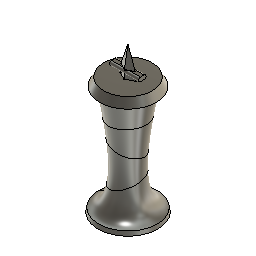
King_v2.4 (Autodesk Fusion 360 design; units mm, degrees)
Autodesk Fusion 360 part; units mm, degrees
sketch "Sketch1" plane through (0, 0, 0) normal (0, 1, 0) x (1, 0, 0)
  spline S0 degree 5 poles (-36.0949, 0) (-34.6298, -0.4528) (-31.8391, -1.6025) (-28.072, -4.0591) (-23.9013, -8.8233) (-20.1701, -17.3686) (-17.9602, -28.572) (-17.1934, -42.2972) (-17.719, -58.2807) (-19.3724, -76.2348) (-22.0047, -95.8993) (-24.8041, -112.843) (-27.2642, -126.1805) (-29.0618, -135.3476) (-30, -140) knots 0 0 0 0 0 0 0.1 0.2 0.3 0.4 0.5 0.6 0.7 0.8 0.9 1 1 1 1 1 1
  line L0 (-30, -140) -> (0, -140)
  line L1 (0, -140) -> (0, 0)
  line L2 (0, 0) -> (-36.0949, 0)
  line L3 (-30, -140) -> (-35.0022, -129.9955)
  line L4 (-35.0022, -129.9955) -> (-28.0309, -129.9955)
  point P0 (-20, -20)
  constraint horizontal L0
  constraint coincident L1.end L2.start
  constraint perpendicular L0 L1
  constraint perpendicular L1 L2
  constraint coincident S0 L4.end
  constraint horizontal L4
revolve "Revolve1" add sketch "Sketch1" angle 360 about axis through (0, 0, 140) along (0, 0, -1) makes body 1
sketch "Sketch2" plane through (0, 0, 140) normal (0, 0, 1) x (-1, 0, 0)
  circle A0 centre (0, 0) radius 30
  line L0 (10, -5) -> (-10, -5)
  line L1 (-10, -5) -> (-10, 5)
  line L2 (-10, 5) -> (10, 5)
  line L3 (10, 5) -> (10, -5)
  line L4 (10, -5) -> (-10, 5) construction
  line L5 (-10, -5) -> (10, 5) construction
  line L6 (10, 0) -> (0, -5)
  line L7 (-10, 0) -> (0, -5)
  line L8 (-10, 0) -> (0, 5)
  line L9 (0, 5) -> (10, 0)
  line L10 (-8.882, 0) -> (0, -4.441)
  line L11 (8.882, 0) -> (0, -4.441)
  line L12 (0, 4.441) -> (8.882, 0)
  line L13 (-8.882, 0) -> (0, 4.441)
  dimension "d4" = 0.5
  constraint horizontal L0
  constraint perpendicular L0 L1
  constraint parallel L0 L2
  constraint parallel L1 L3
  constraint coincident L4 A0.centre
  constraint coincident L5 A0.centre
  constraint coincident A0.centre origin
  constraint midpoint L3 L6.start
  constraint midpoint L0 L6.end
  constraint midpoint L1 L7.start
  constraint midpoint L2 L8.end
extrude "Extrude1" cut sketch "Sketch2" against normal blind 125 contours L6 L7 L8 L9 | L10 L11 L12 L13 bodies 1
extrude "Extrude2" add sketch "Sketch2" along normal blind -123 and the other way blind -35 separate body contours L10 L11 L12 L13 makes body 2
sketch "Sketch3" plane through (0, 0, 0) normal (1, 0, 0) x (0, 1, 0)
  line L0 (4.441, 175) -> (4.441, 17)
  line L1 (-4.441, 17) -> (-4.441, 175)
  line L2 (1.941, 145) -> (-2.6118, 145)
  line L3 (-2.6118, 150) -> (1.941, 150)
  line L4 (-5, 140) -> (5, 140)
  arc A0 (4.441, 147.5) -> (1.941, 150) centre (1.941, 147.5) ccw
  arc A1 (1.941, 145) -> (4.441, 147.5) centre (1.941, 147.5) ccw
  arc A2 (-2.6118, 150) -> (-5.1118, 147.5) centre (-2.6118, 147.5) ccw
  arc A3 (-5.1118, 147.5) -> (-2.6118, 145) centre (-2.6118, 147.5) ccw
  point P0 (4.441, 145)
  point P1 (4.441, 150)
  dimension "d16" = 5
  dimension "d17" = 5
  dimension "d18" = 2.5
  dimension "d19" = 2.5
  dimension "d20" = 2.5
  dimension "d21" = 2.5
  constraint horizontal L2
  constraint horizontal L3
  constraint coincident L0 P0
  constraint coincident P1 L3
  constraint tangent L3 A0
  constraint coincident P0 L2
  constraint tangent L2 A1
  constraint coincident A0.start A1.end
  constraint tangent L3 A2
  constraint tangent L2 A3
  constraint coincident A2.end A3.start
  measures "d16" distance of P0 P1
  measures "d17" distance of P0 L4
  measures "d18" radius of A0
  measures "d19" radius of A1
  measures "d20" radius of A2
  measures "d21" radius of A3
extrude "Extrude3" add sketch "Sketch3" along normal mid plane 36 contours L1 L2 L3 A0 A1 A2 A3 | L1 A2 A3 bodies 2
sketch "Sketch4" plane through (0, 0, 0) normal (1, 0, 0) x (0, 1, 0)
chamfer "Chamfer1" distance 3.9 distance2 25 4 edges at (4.441, 2.2205, 175) (4.441, -2.2205, 175) (-4.441, -2.2205, 175) (-4.441, 2.2205, 175) measured on face at (2.9607, 0, 175) measured on face at (2.9607, 0, 175) measured on face at (2.9607, 0, 175) measured on face at (2.9607, 0, 175) on bodies 2
sketch "Sketch5" plane through (0, 0, 0) normal (0, 1, 0) x (1, 0, 0)
  line L0 (25, -100) -> (-25, -95)
  line L1 (-25, -75) -> (25, -60)
  line L2 (-25, -25) -> (25, -40)
extrude "Extrude4" add 1 faces at (-9.7472, 5.4228, 0) along direction (0, 0, -1) blind 5 draft 10 on bodies 1 bodies 1
ref_plane "WorkPlane1" through (0, 0, 97.5) normal (0.099504, 0, -0.995037) x (-0.995037, 0, -0.099504)
ref_plane "WorkPlane2" through (0, 0, 67.5) normal (0.282982, 0.173648, 0.943275) x (0.957826, 0, -0.287348)
ref_plane "WorkPlane3" through (0, 0, 32.5) normal (-0.277557, -0.258819, 0.925189) x (0.957826, 0, 0.287348)
split "Split1" by plane through (0, 0, 97.5) normal (0.099504, 0, -0.995037) and through (0, 0, 67.5) normal (0.282982, 0.173648, 0.943275) bodies 1 makes body 3 at (-6.1134, -23.257, 107.81) makes body 4 at (21.2338, -0.3953, 89.4601)
split "Split2" by plane through (0, 0, 32.5) normal (-0.277557, -0.258819, 0.925189) bodies 1 makes body 5 at (9.9153, -14.5322, 50.0519)
